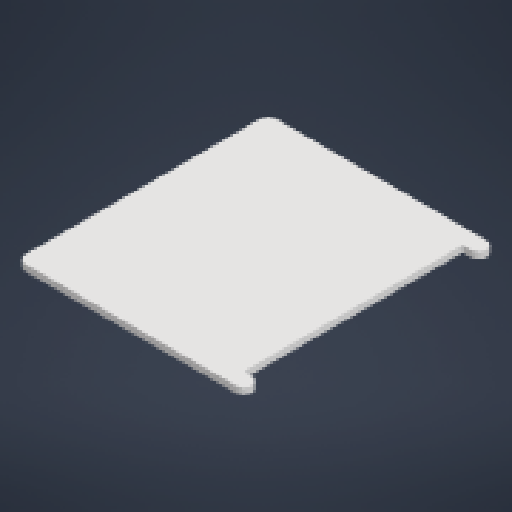
# Autodesk Inventor part: Płytka
Saved by Autodesk Inventor 2025 (Build 290162000, 162)
## iProperties
Created: 2024-04-15
Part Number: Płytka
Material: Generic
Document SubType Name: Modeling
Designer: sicia
Density: 1 g/cm^3
Appearance: Default
Author: sicia
Autodesk Inventor part; units mm, degrees
ref_plane "YZ Plane" through (0, 0, 0) normal (1, 0, 0) x (0, 1, 0)
ref_plane "XZ Plane" through (0, 0, 0) normal (0, 1, 0) x (-1, 0, 0)
ref_plane "XY Plane" through (0, 0, 0) normal (0, 0, 1) x (1, 0, 0)
sketch "Sketch1" plane through (0, 0, 0) normal (0, 1, 0) x (-1, 0, 0)
  line L0 (-10.4167, 14.023) -> (-62.4167, 14.023)
  line L1 (-62.4167, 14.023) -> (-62.4167, -47.977)
  line L2 (-62.4167, -47.977) -> (-10.4167, -47.977)
  line L3 (-10.4167, -47.977) -> (-10.4167, 14.023)
  circle A0 centre (-64.4167, -45.977) radius 2
  line L4 (-64.4167, -43.977) -> (-62.4167, -43.977)
  line L5 (-64.4167, -47.977) -> (-62.4167, -47.977)
  circle A1 centre (-12.4167, 12.023) radius 2
  circle A2 centre (-12.4167, -45.977) radius 2
  circle A3 centre (-64.4167, 12.023) radius 2
  line L6 (-64.4167, 14.023) -> (-62.4167, 14.023)
  line L7 (-64.4167, 10.023) -> (-62.4167, 10.023)
  point P0 (0, 0)
  point P1 (-10.4167, -45.977)
  point P2 (-10.4167, 12.023)
  point P3 (-12.4167, 14.023)
  point P4 (-12.4167, -47.977)
  dimension "d0" = 52
  dimension "d1" = 62
  dimension "d2" = 4
  dimension "d3" = 2
  dimension "d4" = 2
  dimension "d5" = 4
  dimension "d6" = 4
  dimension "d7" = 4
  dimension "d8" = 2
  dimension "d9" = 2
  constraints: 16 end point, 8 tangent, 4 centre point, 4 point on circle, 3 perpendicular, 2 parallel, 2 point on line, 1 horizontal
  measures "d0" distance of L2.end L1.end
  measures "d1" distance of L1.end L0.end
  measures "d2" diameter of A0
  measures "d3" distance from line of L1 A0.centre
  measures "d4" distance from line of L2 A0.centre
  measures "d5" diameter of A1
  measures "d6" diameter of A2
  measures "d7" diameter of A3
  measures "d8" distance from line of L1 A3.centre
  measures "d9" distance from line of L0 A3.centre
extrude "Extrusion1" add sketch "Sketch1" along normal blind 1.6 contours A1 L3 A2 L2 L1 L0 | A1 | L1 A3 L6 | A2 | A3 | L1 L7 A3 | L5 A0 L1 | L1 A0 L4 | A0
body "Solid1"
